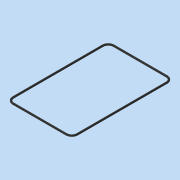
# Autodesk Inventor part: BatteryCaseORing
Saved by Autodesk Inventor 2017 (Build 210142000, 142)
## iProperties
Created: 2018-02-14
Part Number: BatteryCaseORing
Material: Rubber, Silicone
Document SubType Name: Modeling
Designer: Derek Wider
Density: 1.25 g/cm^3
Appearance: Rubber - Black
Author: Derek Wider
Autodesk Inventor part; units mm, degrees
ref_plane "YZ Plane" through (0, 0, 0) normal (1, 0, 0) x (0, 1, 0)
ref_plane "XZ Plane" through (0, 0, 0) normal (0, 1, 0) x (-1, 0, 0)
ref_plane "XY Plane" through (0, 0, 0) normal (0, 0, 1) x (1, 0, 0)
sketch "Sketch2" plane through (0, 0, 0) normal (0, 0, 1) x (1, 0, 0)
  circle A0 centre (0, 0) radius 0.7937
  dimension "d0" = 1.5875
  constraints: 1 centre point, 1 coincident
  measures "d0" diameter of A0
sketch "Sketch3" plane through (0, 0, 0) normal (0, 1, 0) x (-1, 0, 0)
  line L0 (4.7625, 4.7625) -> (52.07, 4.7625)
  line L1 (56.8325, 0) -> (56.8325, -79.6925)
  line L2 (52.07, -84.455) -> (4.7625, -84.455)
  line L3 (0, -79.6925) -> (0, 0)
  arc A0 (56.8325, 0) -> (52.07, 4.7625) centre (52.07, 0) ccw
  arc A1 (52.07, -84.455) -> (56.8325, -79.6925) centre (52.07, -79.6925) ccw
  arc A2 (0, -79.6925) -> (4.7625, -84.455) centre (4.7625, -79.6925) ccw
  arc A3 (4.7625, 4.7625) -> (0, 0) centre (4.7625, 0) ccw
  dimension "d1" = 4.7625
  dimension "d2" = 89.2175
  dimension "d3" = 56.8325
  constraints: 8 end point, 8 point on circle, 8 tangent, 4 centre point, 3 equal radius, 3 perpendicular, 1 coincident, 1 horizontal
  measures "d1" radius of A0
  measures "d2" distance between parallel lines of L2 L0
  measures "d3" distance between parallel lines of L3 L1
sweep "Sweep1" add profiles "Sketch2" path "Sketch3"
body "Solid1"
